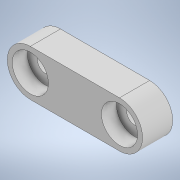
# Autodesk Inventor part: Tope
Saved by Autodesk Inventor 2022 (Build 260153000, 153)
## iProperties
Created: 2021-11-03
Part Number: Tope
Material: Generic
Document SubType Name: Modeling
Designer: juanp
Density: 1 g/cm^3
Appearance: Default
Author: juanp
Autodesk Inventor part; units mm, degrees
ref_plane "YZ Plane" through (0, 0, 0) normal (1, 0, 0) x (0, 1, 0)
ref_plane "XZ Plane" through (0, 0, 0) normal (0, 1, 0) x (-1, 0, 0)
ref_plane "XY Plane" through (0, 0, 0) normal (0, 0, 1) x (1, 0, 0)
sketch "Sketch1" plane through (0, 0, 0) normal (0, 0, 1) x (1, 0, 0)
  line L0 (0, 0) -> (29.6, 0) construction
  line L1 (0, -7.65) -> (29.6, -7.65)
  line L2 (29.6, 7.65) -> (0, 7.65)
  arc A0 (0, 7.65) -> (0, -7.65) centre (0, 0) ccw
  arc A1 (29.6, -7.65) -> (29.6, 7.65) centre (29.6, 0) ccw
  circle A2 centre (0, 0) radius 2.65
  circle A3 centre (29.6, 0) radius 2.65
  point P0 (14.8, 0)
  dimension "d0" = 29.6
  dimension "d1" = 5.3
  dimension "d2" = 5.3
  dimension "d3" = 5
  constraints: 8 end point, 4 centre point, 4 point on circle, 4 tangent, 2 coincident, 1 horizontal, 1 midpoint, 1 parallel
  measures "d0" distance of L0.start L0.end
  measures "d1" diameter of A2
  measures "d2" diameter of A3
  measures "d3" radial gap between concentric circles of A1 A3
extrude "Extrusion1" add sketch "Sketch1" along normal blind 10
sketch "Sketch2" plane through (0, 0, 10) normal (0, 0, 1) x (1, 0, 0)
  circle A0 centre (0, 0) radius 2.65 projected
  circle A1 centre (29.6, 0) radius 2.65 projected
  circle A2 centre (0, 0) radius 6
  circle A3 centre (29.6, 0) radius 6
  dimension "d6" = 12
  constraints: 2 centre point, 2 coincident, 1 equal radius
  measures "d6" diameter of A2
extrude "Extrusion2" cut sketch "Sketch2" against normal blind 5
body "Solid1"
